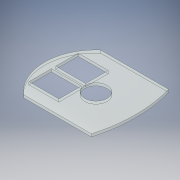
# Autodesk Inventor part: Frame 1
Saved by Autodesk Inventor 2017 (Build 210142000, 142)
## iProperties
Created: 2017-05-26
Part Number: Frame 1
Material: Glass
Document SubType Name: Modeling
Designer: anirudh
Density: 2.18 g/cm^3
Appearance: Clear
Author: anirudh
Autodesk Inventor part; units mm, degrees
ref_plane "YZ Plane" through (0, 0, 0) normal (1, 0, 0) x (0, 1, 0)
ref_plane "XZ Plane" through (0, 0, 0) normal (0, 1, 0) x (-1, 0, 0)
ref_plane "XY Plane" through (0, 0, 0) normal (0, 0, 1) x (1, 0, 0)
sketch "Sketch1" plane through (0, 0, 0) normal (0, 1, 0) x (-1, 0, 0)
  line L0 (0, 180) -> (-158.7451, 180)
  line L1 (0, 180) -> (158.7451, 180)
  line L2 (0, -180) -> (158.7451, -180)
  line L3 (0, -180) -> (-158.7451, -180)
  circle A0 centre (0, 0) radius 52.5
  line L4 (197.8461, 10) -> (57.8461, 10)
  line L5 (57.8461, 10) -> (57.8461, 115)
  line L6 (57.8461, 115) -> (197.8461, 115)
  line L7 (197.8461, 115) -> (197.8461, 10)
  line L8 (197.8461, -10) -> (57.8461, -10)
  line L9 (57.8461, -10) -> (57.8461, -115)
  line L10 (57.8461, -115) -> (197.8461, -115)
  line L11 (197.8461, -115) -> (197.8461, -10)
  arc A1 (-158.7451, 180) -> (-158.7451, -180) centre (466.3502, 0) ccw
  arc A2 (158.7451, -180) -> (158.7451, 180) centre (0, 0) ccw
  dimension "d12" = 105
  dimension "d20" = 140
  dimension "d21" = 105
  dimension "d22" = 140
  dimension "d23" = 105
  constraints: 24 end point, 5 parallel, 4 point on circle, 3 centre point, 3 horizontal, 2 coincident, 2 perpendicular, 2 point on line
  measures "d12" diameter of A0
  measures "d20" distance of L5.end L6.end
  measures "d21" distance of L4.end L5.end
  measures "d22" distance of L10.end L9.end
  measures "d23" distance of L9.end L8.end
extrude "Extrusion1" add sketch "Sketch1" along normal blind 12.7
body "Solid2"
